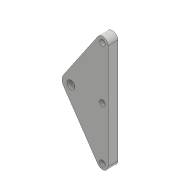
# Autodesk Inventor part: Espacador_Delta
Saved by Autodesk Inventor 2018 (Build 220112000, 112)
## iProperties
Created: 2021-04-28
Part Number: Espacador_Delta
Material: Generic
Document SubType Name: Modeling
Designer: l01767
Density: 1 g/cm^3
Appearance: Default
Author: l01767
Autodesk Inventor part; units mm, degrees
ref_plane "YZ Plane" through (0, 0, 0) normal (1, 0, 0) x (0, 1, 0)
ref_plane "XZ Plane" through (0, 0, 0) normal (0, 1, 0) x (-1, 0, 0)
ref_plane "XY Plane" through (0, 0, 0) normal (0, 0, 1) x (1, 0, 0)
sketch "Sketch1" plane through (0, 0, 0) normal (0, 1, 0) x (-1, 0, 0)
  circle A0 centre (0, 0) radius 18
  line L0 (33.054, 22.5263) -> (-121.3412, 249.0789)
  line L1 (-167, 235) -> (-167, 75.4136)
  circle A1 centre (-142, 235) radius 12.5
  circle A2 centre (-142, 0) radius 12.5
  line L2 (0, 0) -> (-142, 0)
  line L3 (33.054, -22.5263) -> (-121.3412, -249.0789)
  line L4 (-167, -235) -> (-167, 75.4136)
  circle A3 centre (-142, -235) radius 12.5
  arc A4 (-121.3412, 249.0789) -> (-167, 235) centre (-142, 235) ccw
  arc A5 (33.054, -22.5263) -> (33.054, 22.5263) centre (0, 0) ccw
  arc A6 (-167, -235) -> (-121.3412, -249.0789) centre (-142, -235) ccw
  point P0 (-167, 316.0765)
  point P1 (-167, -316.0765)
  dimension "d0" = 36
  dimension "d1" = 25
  dimension "d2" = 25
  dimension "d4" = 142
  dimension "d6" = 470
  dimension "d9" = 25
  dimension "d10" = 40
  constraints: 10 end point, 7 centre point, 6 point on circle, 6 tangent, 4 point on line, 2 concentric, 2 symmetric about line, 1 coincident, 1 equal radius, 1 horizontal, 1 vertical, 1 vertical alignment, 1 other
  measures "d0" diameter of A0
  measures "d1" diameter of A1
  measures "d2" diameter of A2
  measures "d4" distance of L2.start L2.end
  measures "d6" distance of A3.centre A1.centre
  measures "d9" distance from line of L2.end L4
  measures "d10" radius of A5
extrude "Extrusion1" add sketch "Sketch1" along normal mid plane 44.45
body "Solid1"
